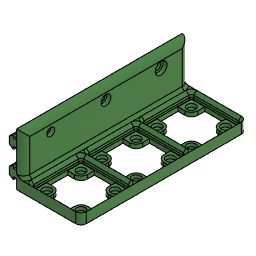
Gridfinity Ender Side Mount (Autodesk Fusion 360 design; units mm, degrees)
Autodesk Fusion 360 part; units mm, degrees
sketch "Gridfinity Base" plane through (0, 0, 0) normal (0, 0, 1) x (1, 0, 0) in component "Gridfinity Baseplate v3"
  line L0 (13, -13) -> (-13, -13) construction
  line L1 (-13, -13) -> (-13, 13) construction
  line L2 (-13, 13) -> (13, 13) construction
  line L3 (13, 13) -> (13, -13) construction
  line L4 (13, -13) -> (-13, 13) construction
  line L5 (-13, -13) -> (13, 13) construction
  line L6 (17, -21) -> (-17, -21)
  line L7 (-21, -17) -> (-21, 17)
  line L8 (-17, 21) -> (17, 21)
  line L9 (21, 17) -> (21, -17)
  line L10 (21, -21) -> (-21, 21) construction
  line L11 (-21, -21) -> (21, 21) construction
  circle A0 centre (13, 13) radius 1.5
  circle A1 centre (13, 13) radius 3.25
  circle A2 centre (13, -13) radius 1.5
  circle A3 centre (13, -13) radius 3.25
  circle A4 centre (-13, -13) radius 1.5
  circle A5 centre (-13, -13) radius 3.25
  circle A6 centre (-13, 13) radius 1.75
  circle A7 centre (-13, 13) radius 3.25
  arc A8 (-17, 21) -> (-21, 17) centre (-17, 17) ccw
  arc A9 (21, 17) -> (17, 21) centre (17, 17) ccw
  arc A10 (17, -21) -> (21, -17) centre (17, -17) ccw
  arc A11 (-21, -17) -> (-17, -21) centre (-17, -17) ccw
  circle A12 centre (-13, -13) radius 5
  circle A13 centre (13, -13) radius 5
  circle A14 centre (-13, 13) radius 5
  circle A15 centre (13, 13) radius 5
  line L12 (21, -8) -> (13, -8)
  line L13 (8, -21) -> (8, -13)
  line L14 (-8, -21) -> (-8, -13)
  line L15 (-21, -8) -> (-13, -8)
  line L16 (21, 8) -> (13, 8)
  line L17 (8, 21) -> (8, 13)
  line L18 (-8, 21) -> (-8, 13)
  line L19 (-21, 8) -> (-13, 8)
  line L20 (18.15, 18.15) -> (-18.15, 18.15)
  line L21 (-18.15, 18.15) -> (-18.15, -18.15)
  line L22 (-18.15, -18.15) -> (18.15, -18.15)
  line L23 (18.15, -18.15) -> (18.15, 18.15)
  line L24 (18.15, 18.15) -> (-18.15, -18.15) construction
  line L25 (-18.15, 18.15) -> (18.15, -18.15) construction
  dimension "d1" = 26
  dimension "d2" = 26
  dimension "d3" = 42
  dimension "d4" = 42
  dimension "d5" = 3
  dimension "d6" = 6.5
  dimension "d7" = 3
  dimension "d8" = 6.5
  dimension "d9" = 3
  dimension "d10" = 6.5
  dimension "d11" = 3.5
  dimension "d12" = 6.5
  dimension "d13" = 4
  dimension "d27" = 10
  dimension "d28" = 10
  dimension "d29" = 10
  dimension "d30" = 10
  dimension "d35" = 36.3
  dimension "d36" = 36.3
  constraint horizontal L0
  constraint perpendicular L0 L1
  constraint parallel L0 L2
  constraint parallel L1 L3
  constraint coincident L4 origin
  constraint coincident L5 origin
  constraint horizontal L6
  constraint perpendicular L6 L7
  constraint parallel L6 L8
  constraint parallel L7 L9
  constraint coincident L10 origin
  constraint coincident L11 origin
  constraint coincident L2.end L3.start
  constraint concentric A0 A1
  constraint coincident L0.start L3.end
  constraint concentric A2 A3
  constraint coincident L0.end L1.start
  constraint concentric A4 A5
  constraint coincident L1.end L2.start
  constraint concentric A6 A7
  constraint coincident L10.end L7
  constraint coincident L10.end L8
  constraint tangent L7 A8
  constraint tangent L8 A8
  constraint coincident L11.end L8
  constraint coincident L11.end L9
  constraint tangent L8 A9
  constraint tangent L9 A9
  constraint equal A8 A9
  constraint coincident L10.start L9
  constraint coincident L10.start L6
  constraint tangent L9 A10
  constraint tangent L6 A10
  constraint equal A8 A10
  constraint coincident L11.start L6
  constraint coincident L11.start L7
  constraint tangent L6 A11
  constraint tangent L7 A11
  constraint equal A8 A11
  constraint concentric A5 A12
  constraint concentric A3 A13
  constraint concentric A7 A14
  constraint concentric A1 A15
  constraint coincident L9 L12.start
  constraint perpendicular L3 L12
  constraint coincident L6 L13.start
  constraint perpendicular L0 L13
  constraint tangent A13 L12
  constraint coincident L3 L12.end
  constraint coincident A13 L13.end
  constraint tangent A13 L13
  constraint coincident L6 L14.start
  constraint perpendicular L0 L14
  constraint coincident L7 L15.start
  constraint perpendicular L1 L15
  constraint coincident L9 L16.start
  constraint perpendicular L3 L16
  constraint coincident L8 L17.start
  constraint perpendicular L2 L17
  constraint coincident L8 L18.start
  constraint perpendicular L2 L18
  constraint coincident L7 L19.start
  constraint perpendicular L1 L19
  constraint coincident A12 L14.end
  constraint coincident A12 L15.end
  constraint coincident A14 L19.end
  constraint coincident A14 L18.end
  constraint coincident A15 L17.end
  constraint coincident A15 L16.end
  constraint tangent A12 L14
  constraint tangent A12 L15
  constraint tangent A14 L19
  constraint tangent A14 L18
  constraint tangent A15 L17
  constraint tangent A15 L16
  constraint horizontal L20
  constraint perpendicular L20 L21
  constraint parallel L20 L22
  constraint parallel L21 L23
  constraint coincident L24 origin
  constraint coincident L25 origin
  measures "d1" distance of L1.end L2.end
  measures "d2" distance of L0.end L1.end
  measures "d3" distance of L10.end L11.end
  measures "d4" distance of L11.start L10.end
  measures "d5" diameter of A0
  measures "d6" diameter of A1
  measures "d7" diameter of A2
  measures "d8" diameter of A3
  measures "d9" diameter of A4
  measures "d10" diameter of A5
  measures "d11" diameter of A6
  measures "d12" diameter of A7
  measures "d13" radius of A8
  measures "d27" diameter of A12
  measures "d28" diameter of A13
  measures "d29" diameter of A14
  measures "d30" diameter of A15
  measures "d35" distance of L21.end L22.end
  measures "d36" distance of L20.end L21.end
sketch "Gridfinity Cross-Section" plane through (0, 0, 0) normal (0, 1, 0) x (1, 0, 0) in component "Gridfinity Baseplate v3"
  line L0 (-21, -5) -> (21, -5)
  line L1 (21, -5) -> (21, 0)
  line L2 (21, 0) -> (-21, 0)
  line L3 (-21, 0) -> (-21, -5)
  line L4 (21, -5) -> (18.85, -2.85)
  line L5 (21, -5) -> (17.4645, -5) construction
  line L6 (18.85, -2.85) -> (18.85, -1.05)
  line L7 (18.85, -1.05) -> (18.15, -0.35)
  line L8 (18.85, -1.05) -> (17.5557, -1.05) construction
  line L9 (0, -5) -> (0, 0)
  line L10 (18.15, -0.35) -> (18.15, 0)
  dimension "d14" = 42
  dimension "d15" = 5
  dimension "d16" = 45
  dimension "d17" = 2.15
  dimension "d18" = 1.8
  dimension "d19" = 45
  dimension "d20" = 0.7
  constraint horizontal L0
  constraint vertical L1
  constraint horizontal L2
  constraint vertical L3
  constraint midpoint L9.end L2
  constraint horizontal L5
  constraint perpendicular L0 L6
  constraint horizontal L8
  constraint midpoint L0 L9.start
  constraint coincident L9.end origin
  constraint coincident L2 L10.end
  constraint perpendicular L2 L10
  measures "d14" distance of L0.start L0.end
  measures "d15" distance of L0.start L2.end
  measures "d16" angle of L4 L5
  measures "d17" vertical distance of L0.end L4.end
  measures "d18" distance of L4.end L6.end
  measures "d19" angle of L7 L8
  measures "d20" vertical distance of L6.end L7.end
sweep "Gridfinity Baseplate" add profiles "Gridfinity Cross-Section" path "Gridfinity Base" along A10 L6 A11 L7 A8 L8 A9 L9 section 1 contours L1 L2 L4 L6 L7 L10 makes body 1 in component "Gridfinity Baseplate v3"
extrude "Magnet Base" add sketch "Gridfinity Base" against normal blind 3 contours L6 L9 A10 L12 L13 L22 L23 | L6 L13 L14 L22 | L6 L7 A11 L14 L15 L21 L22 | A13 L12 L13 L22 L23 | L9 L12 L16 L23 | A12 L14 L15 L21 L22 | A13 | L8 L9 A9 L16 L17 L20 L23 | A12 | A15 L16 L17 L20 L23 | L7 L15 L19 L21 | A15 | L7 L8 A8 L18 L19 L20 L21 | A14 L18 L19 L20 L21 | L8 L17 L18 L20 | A14 | A0 | A1 | A2 | A3 | A4 | A5 | A6 | A7 bodies 1 in component "Gridfinity Baseplate v3"
extrude "Magnet Hole" cut sketch "Gridfinity Base" against normal blind 2.5 contours A0 | A1 | A2 | A3 | A4 | A5 | A6 | A7 bodies 1 in component "Gridfinity Baseplate v3"
copy_body "CopyPasteBodies1" bodies 1 makes body 2 in component "Gridfinity Baseplate v3"
move_body "Move1" bodies 2 to x (1, 0, 0) y (0, 1, 0) z (0, 0, 1) at (0, -42, 0) in component "Gridfinity Baseplate v3"
copy_body "CopyPasteBodies2" bodies 1 makes body 3 in component "Gridfinity Baseplate v3"
move_body "Move2" bodies 3 to x (1, 0, 0) y (0, 1, 0) z (0, 0, 1) at (0, 42, 0) in component "Gridfinity Baseplate v3"
combine "Gridfinity Baseplate Combine" operation add target body 1 tool bodies 2 3 in component "Gridfinity Baseplate v3"
sketch "Gridfinity Baseplate Combine" plane through (0, 0, -3) normal (0, 0, -1) x (1, 0, 0) in component "Gridfinity Baseplate v3"
  line L0 (-8, -29) -> (-8, -23.85)
  line L1 (-8, -23.85) -> (8, -23.85)
  line L2 (8, -23.85) -> (8, -29)
  arc A0 (8, -29) -> (13, -34) centre (13, -29) ccw
  line L3 (13, -34) -> (18.15, -34)
  line L4 (18.15, -34) -> (18.15, -50)
  line L5 (18.15, -50) -> (13, -50)
  arc A1 (13, -50) -> (8, -55) centre (13, -55) ccw
  line L6 (8, -55) -> (8, -60.15)
  line L7 (8, -60.15) -> (-8, -60.15)
  line L8 (-8, -60.15) -> (-8, -55)
  arc A2 (-8, -55) -> (-13, -50) centre (-13, -55) ccw
  line L9 (-13, -50) -> (-18.15, -50)
  line L10 (-18.15, -50) -> (-18.15, -34)
  line L11 (-18.15, -34) -> (-13, -34)
  arc A3 (-13, -34) -> (-8, -29) centre (-13, -29) ccw
  line L12 (-8, 55) -> (-8, 60.15)
  line L13 (-8, 60.15) -> (8, 60.15)
  line L14 (8, 60.15) -> (8, 55)
  arc A4 (8, 55) -> (13, 50) centre (13, 55) ccw
  line L15 (13, 50) -> (18.15, 50)
  line L16 (18.15, 50) -> (18.15, 34)
  line L17 (18.15, 34) -> (13, 34)
  arc A5 (13, 34) -> (8, 29) centre (13, 29) ccw
  line L18 (8, 29) -> (8, 23.85)
  line L19 (8, 23.85) -> (-8, 23.85)
  line L20 (-8, 23.85) -> (-8, 29)
  arc A6 (-8, 29) -> (-13, 34) centre (-13, 29) ccw
  line L21 (-13, 34) -> (-18.15, 34)
  line L22 (-18.15, 34) -> (-18.15, 50)
  line L23 (-18.15, 50) -> (-13, 50)
  arc A7 (-13, 50) -> (-8, 55) centre (-13, 55) ccw
  line L24 (-8, 13) -> (-8, 18.15)
  line L25 (-8, 18.15) -> (8, 18.15)
  line L26 (8, 18.15) -> (8, 13)
  arc A8 (8, 13) -> (13, 8) centre (13, 13) ccw
  line L27 (13, 8) -> (18.15, 8)
  line L28 (18.15, 8) -> (18.15, -8)
  line L29 (18.15, -8) -> (13, -8)
  arc A9 (13, -8) -> (8, -13) centre (13, -13) ccw
  line L30 (8, -13) -> (8, -18.15)
  line L31 (8, -18.15) -> (-8, -18.15)
  line L32 (-8, -18.15) -> (-8, -13)
  arc A10 (-8, -13) -> (-13, -8) centre (-13, -13) ccw
  line L33 (-13, -8) -> (-18.15, -8)
  line L34 (-18.15, -8) -> (-18.15, 8)
  line L35 (-18.15, 8) -> (-13, 8)
  arc A11 (-13, 8) -> (-8, 13) centre (-13, 13) ccw
  arc A12 (-21, -17) -> (-17, -21) centre (-17, -17) ccw
  arc A13 (-17, -21) -> (-21, -25) centre (-17, -25) ccw
  line L36 (-21, -25) -> (-21, -59)
  arc A14 (-21, -59) -> (-17, -63) centre (-17, -59) ccw
  line L37 (-17, -63) -> (17, -63)
  arc A15 (17, -63) -> (21, -59) centre (17, -59) ccw
  line L38 (21, -59) -> (21, -25)
  arc A16 (21, -25) -> (17, -21) centre (17, -25) ccw
  arc A17 (17, -21) -> (21, -17) centre (17, -17) ccw
  line L39 (21, -17) -> (21, 17)
  arc A18 (21, 17) -> (17, 21) centre (17, 17) ccw
  arc A19 (17, 21) -> (21, 25) centre (17, 25) ccw
  line L40 (21, 25) -> (21, 59)
  arc A20 (21, 59) -> (17, 63) centre (17, 59) ccw
  line L41 (17, 63) -> (-17, 63)
  arc A21 (-17, 63) -> (-21, 59) centre (-17, 59) ccw
  line L42 (-21, 59) -> (-21, 25)
  arc A22 (-21, 25) -> (-17, 21) centre (-17, 25) ccw
  arc A23 (-17, 21) -> (-21, 17) centre (-17, 17) ccw
  line L43 (-21, 17) -> (-21, -17)
  line L44 (-21, 63) -> (21, 63)
  line L45 (21, 63) -> (21, -63)
  line L46 (21, -63) -> (-21, -63)
  line L47 (-21, -63) -> (-21, 63)
  line L48 (-21, 63) -> (21, -63) construction
  line L49 (21, 63) -> (-21, -63) construction
  dimension "d37" = 42
  dimension "d38" = 126
  constraint horizontal L44
  constraint perpendicular L44 L45
  constraint parallel L44 L46
  constraint parallel L45 L47
  constraint coincident L48 origin
  constraint coincident L49 origin
  measures "d37" distance of L45.end L46.end
  measures "d38" distance of L44.end L45.end
extrude "Gridfinity Baseplate Combine (1)" add sketch "Gridfinity Baseplate Combine" against normal up to surface (8 mm away) contours A12 A13 L47 | A22 A23 L47 | A14 L46 L47 | A21 L44 L47 | A16 A17 L45 | A18 A19 L45 bodies 1 in component "Gridfinity Baseplate v3"
copy_body "CutPasteBodies1" bodies 1 removing the originals makes body 4
sketch "V Slot Profile" plane through (0, -63, 0) normal (0, -1, 0) x (1, 0, 0)
  line L0 (-23, -3) -> (-28, -3)
  line L1 (-28, -3) -> (-28, 37)
  line L2 (-28, 37) -> (-23, 37)
  line L3 (-23, 37) -> (-23, -3)
  line L4 (-33.5, 9.75) -> (-33.5, 4.25)
  line L5 (-30.5, 2.25) -> (-33.5, 4.25)
  line L6 (-30.5, 4.25) -> (-30.5, 2.25)
  line L7 (-30.5, 4.25) -> (-33.5, 4.25) construction
  line L8 (-30.5, 9.75) -> (-30.5, 11.75)
  line L9 (-30.5, 11.75) -> (-33.5, 9.75)
  line L10 (-30.5, 9.75) -> (-33.5, 9.75) construction
  line L11 (-28, 4.25) -> (-28, 9.75)
  line L12 (-28, 4.25) -> (-30.5, 4.25)
  line L13 (-28, 9.75) -> (-30.5, 9.75)
  line L14 (-28, 27) -> (-28, 7) construction
  line L15 (-30.5, 24.25) -> (-30.5, 22.25)
  line L16 (-33.5, 29.75) -> (-33.5, 24.25)
  line L17 (-30.5, 22.25) -> (-33.5, 24.25)
  line L18 (-28, 24.25) -> (-30.5, 24.25)
  line L19 (-30.5, 24.25) -> (-33.5, 24.25) construction
  line L20 (-30.5, 29.75) -> (-33.5, 29.75) construction
  line L21 (-28, 29.75) -> (-30.5, 29.75)
  line L22 (-30.5, 31.75) -> (-33.5, 29.75)
  line L23 (-30.5, 29.75) -> (-30.5, 31.75)
  line L24 (-28, 24.25) -> (-28, 29.75)
  line L25 (17, -3) -> (17, 5)
  line L26 (17, 5) -> (-17, 5)
  line L27 (-17, 5) -> (-21, 5)
  line L28 (-21, 5) -> (-21, -3)
  line L29 (-21, -3) -> (17, -3)
  line L30 (-21, -3) -> (-23, -3)
  line L31 (-21, 5) -> (-23, 5)
  dimension "d41" = 5
  dimension "d42" = 40
  dimension "d62" = 5.5
  dimension "d63" = 5.5
  dimension "d64" = 2.5
  dimension "d65" = 2
  dimension "d67" = 2.5
  dimension "d68" = 2
  dimension "d49" = 5.5
  dimension "d50" = 20
  dimension "d51" = 5.5
  dimension "d52" = 5.5
  dimension "d53" = 2.5
  dimension "d54" = 2
  dimension "d55" = 2.5
  dimension "d56" = 2
  dimension "d57" = 5.5
  dimension "d101" = 2
  constraint horizontal L0
  constraint vertical L1
  constraint horizontal L2
  constraint vertical L3
  constraint perpendicular L11 L13
  constraint perpendicular L8 L13
  constraint perpendicular L11 L12
  constraint perpendicular L4 L7
  constraint vertical L4
  constraint vertical L11
  constraint vertical L14
  constraint midpoint L1 L14
  constraint perpendicular L21 L24
  constraint perpendicular L21 L23
  constraint perpendicular L18 L24
  constraint perpendicular L16 L19
  constraint vertical L16
  constraint vertical L24
  constraint vertical L15
  constraint vertical L6
  constraint midpoint L11 L14.end
  constraint midpoint L14.start L24
  constraint horizontal L30
  constraint coincident L28.end L29.start
  constraint coincident L27.end L28.start
  constraint coincident L3 L31.end
  constraint perpendicular L3 L31
  measures "d41" distance of L0.end L0.start
  measures "d42" distance of L2.end L0.start
  measures "d62" distance of L11.end L11.start
  measures "d63" distance of L11.start L4.end
  measures "d64" distance of L11.start L6.start
  measures "d65" distance of L5.start L6.start
  measures "d67" distance of L11.end L8.start
  measures "d68" distance of L8.start L8.end
  measures "d49" distance of L4.end L4.start
  measures "d50" distance of L14.start L14.end
  measures "d51" distance of L18.start L21.start
  measures "d52" distance of L16.end L18.start
  measures "d53" distance of L15.start L18.start
  measures "d54" distance of L15.start L15.end
  measures "d55" distance of L20.start L21.start
  measures "d56" distance of L22.start L20.start
  measures "d57" distance of L16.end L16.start
  measures "d101" distance of L28.end L0.start
extrude "V Slot Profile (1)" add sketch "V Slot Profile" against normal up to surface (126 mm away) contours L0 L1 L2 L3 L11 L24 | L3 L28 L30 L31 | L1 L4 L5 L6 L8 L9 L11 L12 L13 | L1 L15 L16 L17 L18 L21 L22 L23 L24 bodies 4
sketch "T Nuts" plane through (-28, 0, 0) normal (-1, 0, 0) x (0, -1, 0)
  line L0 (-63, 24.25) -> (-63, 9.75) construction
  line L1 (-63, 9.75) -> (63, 9.75)
  line L2 (63, 9.75) -> (63, 24.25)
  line L3 (63, 24.25) -> (-63, 24.25)
  line L4 (21, 27) -> (63, 27) construction
  line L5 (63, 27) -> (63, 7) construction
  line L6 (63, 7) -> (21, 7) construction
  line L7 (21, 7) -> (21, 27) construction
  line L8 (-21, 27) -> (21, 27) construction
  line L9 (21, 7) -> (-21, 7) construction
  line L10 (21, 27) -> (21, 7) construction
  line L11 (-21, 7) -> (-21, 27) construction
  line L12 (-21, 7) -> (-63, 7) construction
  line L13 (-63, 7) -> (-63, 27) construction
  line L14 (-63, 27) -> (-21, 27) construction
  line L15 (-21, 27) -> (-21, 7) construction
  circle A0 centre (42, 27) radius 1.675
  circle A1 centre (0, 27) radius 2.25
  circle A2 centre (-42, 27) radius 2.75
  line L16 (-63, 27) -> (-21, 7) construction
  line L17 (-21, 7) -> (21, 27) construction
  line L18 (21, 27) -> (63, 7) construction
  line L19 (10, -3) -> (-10, -3)
  line L20 (-10, -3) -> (-10, 37)
  line L21 (-10, 37) -> (10, 37)
  line L22 (10, 37) -> (10, -3)
  line L23 (10, -3) -> (-10, 37) construction
  line L24 (-10, -3) -> (10, 37) construction
  line L25 (-21, 27) -> (21, 7) construction
  line L26 (-63, 7) -> (-21, 27) construction
  line L27 (21, 7) -> (63, 27) construction
  line L28 (-32, -3) -> (-52, -3)
  line L29 (-52, -3) -> (-52, 37)
  line L30 (-52, 37) -> (-32, 37)
  line L31 (-32, 37) -> (-32, -3)
  line L32 (-32, -3) -> (-52, 37) construction
  line L33 (-52, -3) -> (-32, 37) construction
  line L34 (52, -3) -> (32, -3)
  line L35 (32, -3) -> (32, 37)
  line L36 (32, 37) -> (52, 37)
  line L37 (52, 37) -> (52, -3)
  line L38 (52, -3) -> (32, 37) construction
  line L39 (32, -3) -> (52, 37) construction
  point P0 (0, 17)
  point P1 (-42, 17)
  point P2 (42, 17)
  dimension "d60" = 42
  dimension "d61" = 20
  dimension "d66" = 42
  dimension "d70" = 3.35
  dimension "d71" = 4.5
  dimension "d72" = 5.5
  dimension "d73" = 42
  dimension "d74" = 20
  dimension "d75" = 40
  dimension "d76" = 20
  dimension "d77" = 40
  dimension "d78" = 20
  dimension "d79" = 40
  constraint horizontal L4
  constraint vertical L5
  constraint horizontal L6
  constraint vertical L7
  constraint horizontal L8
  constraint vertical L10
  constraint horizontal L9
  constraint vertical L11
  constraint midpoint L2 L5
  constraint horizontal L12
  constraint vertical L13
  constraint horizontal L14
  constraint vertical L15
  constraint coincident L4.start L7.end
  constraint coincident L8.start L11.end
  constraint midpoint L4 A0.centre
  constraint midpoint L8 A1.centre
  constraint midpoint L14 A2.centre
  constraint midpoint L0 L13
  constraint horizontal L19
  constraint perpendicular L19 L20
  constraint parallel L19 L21
  constraint parallel L20 L22
  constraint coincident L23 P0
  constraint coincident L24 P0
  constraint midpoint L17 P0
  constraint horizontal L28
  constraint perpendicular L28 L29
  constraint parallel L28 L30
  constraint parallel L29 L31
  constraint coincident L32 P1
  constraint coincident L33 P1
  constraint midpoint L26 P1
  constraint horizontal L34
  constraint perpendicular L34 L35
  constraint parallel L34 L36
  constraint parallel L35 L37
  constraint coincident L38 P2
  constraint coincident L39 P2
  constraint midpoint L18 P2
  measures "d60" distance of L4.start L4.end
  measures "d61" distance of L4.start L6.end
  measures "d66" distance of L8.start L4.start
  measures "d70" diameter of A0
  measures "d71" diameter of A1
  measures "d72" diameter of A2
  measures "d73" distance of L13.end L8.start
  measures "d74" distance of L20.end L21.end
  measures "d75" distance of L19.end L20.end
  measures "d76" distance of L29.end L30.end
  measures "d77" distance of L28.end L29.end
  measures "d78" distance of L35.end L36.end
  measures "d79" distance of L34.end L35.end
extrude "T Nuts (1)" cut sketch "T Nuts" along normal up to surface (5.5 mm away) contours L1 L3 L29 L31 | L1 L28 L29 L31 | A2 | L3 L29 L30 L31 | L1 L3 L20 L22 | L1 L19 L20 L22 | L3 L20 L21 L22 | L1 L3 L35 L37 | L1 L34 L35 L37 | L3 L35 L36 L37 | A0 | A1 bodies 4
extrude "T Nut Screws" cut sketch "T Nuts" against normal up to surface (5 mm away) contours A2 | A0 | A1 bodies 4
sketch "T Nut Screws Counterbore" plane through (-23, 0, 0) normal (1, 0, 0) x (0, 1, 0)
  circle A0 centre (42, 27) radius 2.75
  circle A1 centre (0, 27) radius 2.25
  circle A2 centre (-42, 27) radius 1.675
  line L0 (63, 5) -> (63, 37)
  line L1 (63, 37) -> (-63, 37)
  line L2 (-63, 37) -> (-63, 5)
  circle A3 centre (42, 27) radius 4.5
  circle A4 centre (0, 27) radius 3.75
  circle A5 centre (-42, 27) radius 3
  line L3 (-63, 5) -> (63, 5)
  dimension "d84" = 9
  dimension "d85" = 7.5
  dimension "d86" = 6
  constraint concentric A0 A3
  constraint concentric A1 A4
  constraint concentric A2 A5
  measures "d84" diameter of A3
  measures "d85" diameter of A4
  measures "d86" diameter of A5
extrude "T Nut Screws Counterbore (1)" cut sketch "T Nut Screws Counterbore" against normal blind 3 contours A3 | A4 | A5 bodies 4
fillet "Exterior Fillet" radius 5 3 edges at (-23, -63, 21) (-23, 63, 21) (-23, 0, 37) on bodies 4
fillet "Fillet2" radius 2 1 edges at (-23, 0, 5) on bodies 4
ref_plane "WorkPlane1" through (-27, 0, 17) normal (-1, 0, 0) x (0, 0, 1)
sketch "Ljm" plane through (-27, 0, 17) normal (-1, 0, 0) x (0, 1, 0)
  circle A0 centre (0, 4) radius 8
  spline S0 degree 3 poles (-1.051, 6.2614) (-1.051, 6.2615) (-1.0533, 6.6672) (-0.5659, 6.6672) (-0.1002, 6.6672) (-0.0808, 6.263) (-0.0808, 6.263) knots 28 28 28 28 29 29 29 30 30 30 30
  spline S1 degree 3 poles (0.2425, 7.2332) (0.2425, 7.2332) (0.2425, 9.6586) (2.5871, 9.6586) (4.9345, 9.6586) (4.9317, 7.2332) (4.9317, 7.2332) knots 6 6 6 6 7 7 7 8 8 8 8
  spline S2 degree 3 poles (5.4168, -0.1396) (6.3593, 1.0231) (6.8745, 2.5035) (6.8745, 4.1169) (6.8745, 7.8559) (3.8434, 10.887) (0.1044, 10.887) (-2.7686, 10.887) (-5.2219, 9.0964) (-6.205, 6.571) knots 13 13 13 13 14 14 14 15 15 15 16 16 16 16
  spline S3 degree 3 poles (-2.9914, 2.7057) (-2.9914, 2.7057) (-2.5383, 2.3014) (-2.0212, 2.3014) (-1.4523, 2.3014) (-1.051, 2.7057) (-1.051, 2.7057) knots 25 25 25 25 26 26 26 27 27 27 27
  line L0 (-0.0808, 6.263) -> (-0.0808, 1.6706)
  circle A1 centre (0, 4) radius 9.6
  spline S4 degree 3 poles (1.2127, 3.1908) (1.2127, 3.1908) (1.2127, 2.7865) (0.6866, 2.7865) (0.2425, 2.7865) (0.2425, 3.1908) (0.2425, 3.1908) knots 3 3 3 3 4 4 4 5 5 5 5
  spline S5 degree 3 poles (0.7422, 2.0306) (1.0504, 2.0306) (1.3003, 1.7807) (1.3003, 1.4725) (1.3003, 1.1642) (1.0504, 0.9143) (0.7422, 0.9143) (0.4339, 0.9143) (0.1841, 1.1642) (0.1841, 1.4725) (0.1841, 1.7807) (0.4339, 2.0306) (0.7422, 2.0306) knots 0 0 0 0 1 1 1 2 2 2 3 3 3 4 4 4 4
  spline S6 degree 3 poles (5.0934, 6.6672) (5.0934, 6.6672) (5.1774, 6.6731) (5.3128, 6.5377) (5.4184, 6.4321) (5.4168, 6.3439) (5.4168, 6.3439) knots 10 10 10 10 11 11 11 12 12 12 12
  spline S7 degree 3 poles (-0.7953, 0.4043) (-0.7953, 0.4043) (0.8951, 0.4207) (1.9445, 0.0291) (3.2729, -0.4667) (3.9743, -1.4302) (3.9743, -1.4302) knots 1 1 1 1 2 2 2 3 3 3 3
  spline S8 degree 3 poles (-3.7144, 0.6232) (-2.3776, 0.3931) (-0.7953, 0.4043) (-0.7953, 0.4043) knots 0 0 0 0 1 1 1 1
  line L1 (4.4467, 5.6971) -> (1.8595, 5.6971)
  line L2 (0.2425, 3.1908) -> (0.2425, 7.2332)
  line L3 (1.2127, 7.2332) -> (1.2127, 3.1908)
  spline S9 degree 3 poles (-1.051, 1.6406) (-1.051, 1.6406) (-1.3515, 1.3313) (-2.0212, 1.3313) (-3.0737, 1.3313) (-3.4289, 1.9602) (-3.4289, 1.9602) knots 33 33 33 33 34 34 34 35 35 35 35
  ellipse E0 centre (4.4578, 11.7439) end of major axis (13.1952, 24.361) minor radius 8.5701 (-6.2704, 1.8387) -> (-6.0537, 1.3051) ccw
  spline S10 degree 3 poles (1.8595, 5.6971) (1.8595, 5.6971) (1.4553, 5.7054) (1.4553, 6.1846) (1.4553, 6.6536) (1.8595, 6.6672) (1.8595, 6.6672) knots 7 7 7 7 8 8 8 9 9 9 9
  spline S11 degree 3 poles (-5.9019, 2.7057) (-5.9019, 2.7057) (-5.5805, 2.3014) (-4.9326, 2.3014) (-4.1715, 2.3014) (-3.9616, 2.7057) (-3.9616, 2.7057) knots 19 19 19 19 20 20 20 21 21 21 21
  line L4 (-3.9616, 2.7057) -> (-3.9616, 6.263)
  spline S12 degree 3 poles (-3.9616, 6.263) (-3.9616, 6.263) (-3.9095, 6.6672) (-3.4765, 6.6672) (-3.0124, 6.6672) (-2.9914, 6.263) (-2.9914, 6.263) knots 22 22 22 22 23 23 23 24 24 24 24
  line L5 (1.8595, 6.6672) -> (5.0934, 6.6672)
  line L6 (-2.9914, 6.263) -> (-2.9914, 2.7057)
  line L7 (3.9743, -1.4302) -> (3.9835, -1.4302)
  line L8 (5.4168, 6.3439) -> (5.4168, -0.1396)
  spline S13 degree 3 poles (3.9616, 7.2332) (3.9616, 7.2332) (4.0864, 8.6885) (2.5871, 8.6885) (1.1011, 8.6885) (1.2127, 7.2332) (1.2127, 7.2332) knots 0 0 0 0 1 1 1 2 2 2 2
  spline S14 degree 3 poles (-6.205, 6.571) (-6.2022, 6.57) (-6.1059, 6.5349) (-6.04, 6.469) (-5.9137, 6.3427) (-5.9019, 6.263) (-5.9019, 6.263) knots 16 16 16 16 17 17 17 18 18 18 18
  line L9 (-5.9019, 6.263) -> (-5.9019, 2.7057)
  line L10 (4.4467, -1.0355) -> (4.4467, 5.6971)
  spline S15 degree 3 poles (-3.4289, 1.9602) (-3.4289, 1.9602) (-3.8102, 1.3313) (-4.9317, 1.3313) (-5.895, 1.3313) (-6.1339, 1.7567) (-6.2704, 1.8387) knots 35 35 35 35 36 36 36 37 37 37 37
  spline S16 degree 3 poles (3.9835, -1.4302) (4.1597, -1.3067) (4.2833, -1.1747) (4.4467, -1.0355) knots 4 4 4 4 5 5 5 5
  line L11 (-1.051, 2.7057) -> (-1.051, 6.2614)
  spline S17 degree 3 poles (-0.0808, 1.6706) (-0.0808, 1.6706) (-0.1052, 1.326) (-0.5659, 1.326) (-1.0683, 1.326) (-1.051, 1.6406) (-1.051, 1.6406) knots 31 31 31 31 32 32 32 33 33 33 33
  spline S18 degree 3 poles (-6.0537, 1.3051) (-5.9126, 1.2447) (-4.9186, 0.8306) (-3.7144, 0.6232) knots 38 38 38 38 39 39 39 39
  line L12 (4.9317, 7.2332) -> (3.9616, 7.2332)
  constraint parallel L5 L12
  constraint concentric A0 A1
sketch "Ljm Path" plane through (0, 0, 0) normal (0, 1, 0) x (1, 0, 0)
  line L0 (-30.1199, -15.3925) -> (-37.1909, -22.4636)
  line L1 (-30.1199, -15.3925) -> (-40.1199, -15.3925) construction
  dimension "d93" = 45
  dimension "d94" = 10
  constraint horizontal L1
  measures "d93" angle of L0 L1
  measures "d94" distance of L0.start L0.end
sweep "Ljm (1)" cut profiles "Ljm" path "Ljm Path" along L0 section 1 bodies 4
component "Gridfinity Baseplate v3" placed x (1, 0, 0) y (0, 1, 0) z (0, 0, 1) at (0, 0, 0)
named bodies: "Gridfinity Baseplate", "Gridfinity Baseplate (1)", "Gridfinity Baseplate (1) (1)", "Gridfinity Ender Side Mount"
